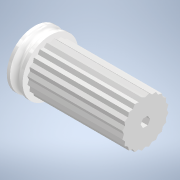
# Autodesk Inventor part: SolidRoller
Saved by Autodesk Inventor 2021 (Build 250183000, 183)
## iProperties
Created: 2021-05-21
Part Number: SolidRoller
Material: PC/ABS Plastic
Document SubType Name: Modeling
Designer: sami8
Density: 0.357273 g/cm^3
Appearance: Smooth - White
Author: sami8
Autodesk Inventor part; units mm, degrees
ref_plane "YZ Plane" through (0, 0, 0) normal (1, 0, 0) x (0, 1, 0)
ref_plane "XZ Plane" through (0, 0, 0) normal (0, 1, 0) x (-1, 0, 0)
ref_plane "XY Plane" through (0, 0, 0) normal (0, 0, 1) x (1, 0, 0)
sketch "Sketch1" plane through (0, 0, 0) normal (1, 0, 0) x (0, 1, 0)
  circle A0 centre (0, 0) radius 14.75 construction
  line L0 (2.6, -1.5011) -> (0, -3.0022)
  line L1 (0, -3.0022) -> (-2.6, -1.5011)
  line L2 (-2.6, -1.5011) -> (-2.6, 1.5011)
  line L3 (-2.6, 1.5011) -> (0, 3.0022)
  line L4 (0, 3.0022) -> (2.6, 1.5011)
  line L5 (2.6, 1.5011) -> (2.6, -1.5011)
  line L6 (14.5684, 2.3074) -> (14.5684, -2.3074) construction
  line L7 (14.5684, 2.3074) -> (0, 0) construction
  line L8 (0, 0) -> (14.5684, -2.3074) construction
  line L9 (14.5684, 2.3074) -> (13.5684, 0)
  line L10 (13.5684, 0) -> (14.5684, -2.3074)
  line L11 (13.5684, 0) -> (14.5684, 0) construction
  line L12 (13.1423, 6.6964) -> (12.9043, 4.1929)
  line L13 (12.9043, 4.1929) -> (14.5684, 2.3074)
  line L14 (10.4298, 10.4298) -> (10.9771, 7.9753)
  line L15 (10.9771, 7.9753) -> (13.1423, 6.6964)
  line L16 (6.6964, 13.1423) -> (7.9753, 10.9771)
  line L17 (7.9753, 10.9771) -> (10.4298, 10.4298)
  line L18 (2.3074, 14.5684) -> (4.1929, 12.9043)
  line L19 (4.1929, 12.9043) -> (6.6964, 13.1423)
  line L20 (-2.3074, 14.5684) -> (0, 13.5684)
  line L21 (0, 13.5684) -> (2.3074, 14.5684)
  line L22 (-6.6964, 13.1423) -> (-4.1929, 12.9043)
  line L23 (-4.1929, 12.9043) -> (-2.3074, 14.5684)
  line L24 (-10.4298, 10.4298) -> (-7.9753, 10.9771)
  line L25 (-7.9753, 10.9771) -> (-6.6964, 13.1423)
  line L26 (-13.1423, 6.6964) -> (-10.9771, 7.9753)
  line L27 (-10.9771, 7.9753) -> (-10.4298, 10.4298)
  line L28 (-14.5684, 2.3074) -> (-12.9043, 4.1929)
  line L29 (-12.9043, 4.1929) -> (-13.1423, 6.6964)
  line L30 (-14.5684, -2.3074) -> (-13.5684, 0)
  line L31 (-13.5684, 0) -> (-14.5684, 2.3074)
  line L32 (-13.1423, -6.6964) -> (-12.9043, -4.1929)
  line L33 (-12.9043, -4.1929) -> (-14.5684, -2.3074)
  line L34 (-10.4298, -10.4298) -> (-10.9771, -7.9753)
  line L35 (-10.9771, -7.9753) -> (-13.1423, -6.6964)
  line L36 (-6.6964, -13.1423) -> (-7.9753, -10.9771)
  line L37 (-7.9753, -10.9771) -> (-10.4298, -10.4298)
  line L38 (-2.3074, -14.5684) -> (-4.1929, -12.9043)
  line L39 (-4.1929, -12.9043) -> (-6.6964, -13.1423)
  line L40 (2.3074, -14.5684) -> (0, -13.5684)
  line L41 (0, -13.5684) -> (-2.3074, -14.5684)
  line L42 (6.6964, -13.1423) -> (4.1929, -12.9043)
  line L43 (4.1929, -12.9043) -> (2.3074, -14.5684)
  line L44 (10.4298, -10.4298) -> (7.9753, -10.9771)
  line L45 (7.9753, -10.9771) -> (6.6964, -13.1423)
  line L46 (13.1423, -6.6964) -> (10.9771, -7.9753)
  line L47 (10.9771, -7.9753) -> (10.4298, -10.4298)
  line L48 (14.5684, -2.3074) -> (12.9043, -4.1929)
  line L49 (12.9043, -4.1929) -> (13.1423, -6.6964)
  dimension "d0" = 29.5
  dimension "d1" = 5.2
  dimension "d2" = 18
  dimension "d3" = 1
  dimension "d6" = 360
  constraints: 100 end point, 2 coincident, 2 point on circle, 2 vertical, 1 centre point, 1 horizontal, 1 midpoint, 114 other
  measures "d0" diameter of A0
  measures "d1" distance between parallel lines of L5 L2
  measures "d2" angle of L8 L7
  measures "d3" distance of L9.end L11.end
extrude "Extrusion1" add sketch "Sketch1" along normal mid plane 70
sketch "Sketch2" plane through (0, 0, 0) normal (0, 0, 1) x (1, 0, 0)
  line L0 (-35, 14.5684) -> (35, 14.5684) projected
  line L1 (-35, -14.5684) -> (35, -14.5684) projected
  line L2 (-35, 14.5684) -> (-25, 14.5684)
  line L3 (-25, 14.5684) -> (-25, -14.5684)
  line L4 (-25, -14.5684) -> (-35, -14.5684)
  line L5 (-35, -14.5684) -> (-35, 14.5684)
  line L6 (-35, 4.5684) -> (-25, 4.5684)
  line L7 (-35, 14.5684) -> (-35, 14.5684)
  line L8 (-35, 14.5684) -> (-33, 14.5684)
  line L9 (-25, 14.5684) -> (-25, 14.5684)
  line L10 (-25, 14.5684) -> (-27, 14.5684)
  arc A0 (-33, 14.5684) -> (-27, 14.5684) centre (-30, 16.3712) ccw
  line L11 (-35, 0) -> (35, 0) projected
  line L12 (-35, 0) -> (-25, 0)
  line L13 (-35, 14.5684) -> (-25, 14.5684)
  line L14 (-25, 14.5684) -> (-25, 20.6242)
  line L15 (-25, 20.6242) -> (-35, 20.6242)
  line L16 (-35, 20.6242) -> (-35, 14.5684)
  point P0 (0, 0)
  dimension "d11" = 0
  dimension "d12" = 10
  dimension "d13" = 10
  dimension "d14" = 2
  dimension "d15" = 0
  dimension "d16" = 2
  dimension "d17" = 0
  dimension "d18" = 3.5
  constraints: 28 end point, 6 point on line, 5 perpendicular, 4 parallel, 2 horizontal, 2 midpoint, 2 point on circle, 2 vertical, 1 centre point, 1 collinear
  measures "d11" distance from line of L0.start L5
  measures "d12" distance of L2.end L2.start
  measures "d13" distance between parallel lines of L0 L6
  measures "d14" distance of L7.end L8.end
  measures "d15" distance of L2.start L7.end
  measures "d16" distance of L9.end L10.end
  measures "d17" distance of L2.end L9.end
  measures "d18" radius of A0
revolve "Revolution2" cut sketch "Sketch2" angle 360 about axis through (-35, 0, 0) along (1, 0, 0) contours L16 L15 L14 L0 | L0 A0 L3 L6 L5 | L0 A0
revolve "Revolution1" add sketch "Sketch2" angle 360 about axis through (-35, 0, 0) along (1, 0, 0) contours L0 A0 L3 L6 L5
body "Solid1"
